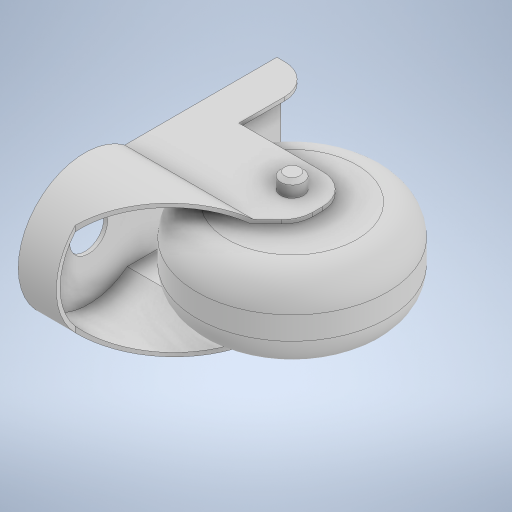
# Autodesk Inventor part: Колесо
Saved by Autodesk Inventor 2023 (Build 270158000, 158)
## iProperties
Created: 2022-04-27
Part Number: Колесо
Material: Типовые
Document SubType Name: Modeling
Designer: User
Density: 1 g/cm^3
Appearance: По умолчанию
Author: User
Autodesk Inventor part; units mm, degrees
ref_plane "YZ Plane" through (0, 0, 0) normal (1, 0, 0) x (0, 1, 0)
sketch "Эскиз1" plane through (0, 0, 0) normal (0, 1, 0) x (-1, 0, 0)
  point P0 (0, 0)
sketch "Эскиз2" plane through (0, 0, 0) normal (0, 1, 0) x (-1, 0, 0)
  line L0 (0, 0) -> (0, -68)
  line L1 (0, -68) -> (-10, -68)
  line L2 (-10, -68) -> (-10, -48)
  line L3 (-10, -48) -> (-40, -48)
  line L4 (0, 0) -> (-10, 0)
  line L5 (-10, 0) -> (-10, -5)
  line L6 (-40, -48) -> (-40, -34)
  line L7 (-40, -34) -> (-10, -5)
  dimension "d0" = 68
  dimension "d1" = 10
  dimension "d2" = 20
  dimension "d3" = 30
  dimension "d4" = 5
  dimension "d5" = 14
  constraints: 16 end point, 3 perpendicular, 2 parallel, 2 point on line, 1 vertical
  measures "d0" distance of L0.start L0.end
  measures "d1" distance of L0.end L1.end
  measures "d2" distance of L1.end L2.end
  measures "d3" distance of L2.end L3.end
  measures "d4" distance of L4.end L5.end
  measures "d5" distance of L3.end L6.end
extrude "Выдавливание1" add sketch "Эскиз2" along normal blind 28
sketch "Эскиз3" plane through (0, 0, -68) normal (-1, 0, 0) x (0, 0, 1)
  line L0 (68, 0) -> (68, 28) projected
  line L1 (68, 14) -> (33, 14)
  arc A0 (40, 0) -> (40, 28) centre (50.5, 14) ccw
  line L2 (0, 0) -> (68, 0) projected
  line L3 (40, 0) -> (0, 0)
  line L4 (20, 28) -> (0, 28) projected
  line L5 (0, 0) -> (0, 28)
  line L6 (0, 28) -> (40, 28)
  line L7 (0, 28) -> (68, 28) projected
  dimension "d8" = 35
  constraints: 8 end point, 3 point on circle, 2 midpoint, 2 point on line, 1 centre point, 1 collinear, 1 horizontal, 1 perpendicular
  measures "d8" distance of L1.start L1.end
extrude "Выдавливание2" add sketch "Эскиз3" against normal blind 40 contours A0 L2 L5 L4 L6 L7 | A0 L2 | L7 A0
ref_plane "РабПлоскость1" through (0, -23.25, 0) normal (0, -1, 0) x (1, 0, 0)
sketch "Эскиз4" plane through (0, -23.25, 0) normal (0, -1, 0) x (1, 0, 0)
  line L0 (0, -68) -> (40, -68) projected
  line L1 (0, -68) -> (10, -68)
  line L2 (10, -68) -> (10, -48)
  line L3 (10, -48) -> (40, -48)
  line L4 (40, -48) -> (40, -34)
  line L5 (10, 0) -> (10, -5) projected
  line L6 (40, -34) -> (10, -5)
  line L7 (0, 0) -> (10, 0) projected
  line L8 (10, -5) -> (10, 0)
  line L9 (10, 0) -> (0, 0)
  line L10 (0, 0) -> (0, -68)
  dimension "d12" = 10
  dimension "d13" = 20
  dimension "d14" = 30
  dimension "d15" = 14
  constraints: 16 end point, 6 perpendicular, 1 point on line
  measures "d12" distance of L0.start L1.end
  measures "d13" distance of L1.end L2.end
  measures "d14" distance of L2.end L3.end
  measures "d15" distance of L3.end L4.end
extrude "Выдавливание3" cut sketch "Эскиз4" against normal blind 139 keep common part
sketch "Эскиз5" plane through (0, 0, 0) normal (-1, 0, 0) x (0, 0, 1)
  arc A0 (-28, 0) -> (-7, 0) centre (-17.5, 14) ccw projected
  circle A1 centre (-17.5, 14) radius 17.5
  line L0 (-68, 0) -> (-68, 28) projected
  line L1 (-28, 0) -> (-68, 0)
  line L2 (-68, 0) -> (-68, 28)
  arc A2 (-7, 28) -> (-28, 28) centre (-17.5, 14) ccw projected
  line L3 (-68, 28) -> (-28, 28)
  point P0 (0, 0)
  constraints: 6 end point, 3 perpendicular, 1 centre point, 1 coincident, 1 point on circle
extrude "Выдавливание4" cut sketch "Эскиз5" against normal blind 43.75 keep common part
sketch "Эскиз6" plane through (40, 0, -34) normal (1, 0, 0) x (0, 0, -1)
  arc A0 (-29, 1.7526) -> (-6, 0) centre (-16.5, 14) ccw projected
  circle A1 centre (-16.5, 14) radius 16.5
  line L0 (0, 0) -> (0, 28) projected
  line L1 (0, 14) -> (34.1975, 14)
  line L2 (34, 28) -> (-6, 28) projected
  line L3 (34, 0) -> (-6, 0) projected
  line L4 (34, 28) -> (34, 0)
  line L5 (34, 0) -> (34, 28) projected
  line L6 (34, 28) -> (34, 27)
  line L7 (34, 27) -> (-6.3388, 27)
  line L8 (34, 0) -> (34, 1)
  line L9 (34, 1) -> (-6.3388, 1)
  line L10 (34, 27) -> (-6.3388, 27)
  line L11 (34, 27) -> (34, 1)
  point P0 (-34, 0)
  point P1 (0, 27)
  dimension "d20" = 33
  dimension "d21" = 1
  dimension "d22" = 1
  constraints: 16 end point, 3 perpendicular, 2 horizontal, 2 point on circle, 2 point on line, 1 centre point, 1 coincident, 1 midpoint
  measures "d20" diameter of A1
  measures "d21" distance of L2.start L6.end
  measures "d22" distance of L3.start L8.end
extrude "Выдавливание5" cut sketch "Эскиз6" against normal blind 39 contours A1 | L0 L9 A1 | L1 L4 L9 L0 | A1 L7 L0 | L0 L7 L4 L1
fillet "Сопряжение1" radius 8 2 edges at (40, 0.5, -48) (40, 27.5, -48)
fillet "Сопряжение2" radius 8 2 edges at (40, 0.5, -34) (40, 27.5, -34)
fillet "Сопряжение3" radius 8 2 edges at (10, 0.5, -68) (10, 27.5, -68)
sketch "Эскиз7" plane through (0, 28, 0) normal (0, 1, 0) x (1, 0, 0)
  arc A0 (40, 40) -> (32, 48) centre (32, 40) ccw projected
  circle A1 centre (32, 40) radius 3
  point P0 (0, 0)
  dimension "d28" = 6
  constraints: 1 centre point, 1 coincident
  measures "d28" diameter of A1
extrude "Выдавливание6" add sketch "Эскиз7" along normal blind 4 and the other way blind 32
sketch "Эскиз8" plane through (1, 0, -34) normal (1, 0, 0) x (0, 0, -1)
  arc A0 (-6.3388, 27) -> (-29, 24.7703) centre (-16.5, 14) ccw projected
  circle A1 centre (-16.5, 14) radius 5
  point P0 (-34, 0)
  dimension "d31" = 10
  constraints: 1 centre point, 1 coincident
  measures "d31" diameter of A1
extrude "Выдавливание7" cut sketch "Эскиз8" against normal blind 31
ref_plane "РабПлоскость2" through (1, 3, -27.6612) normal (0, 1, 0) x (1, 0, 0)
sketch "Эскиз9" plane through (1, 3, -27.6612) normal (0, 1, 0) x (1, 0, 0)
  circle A0 centre (31, 12.3388) radius 3 projected
  circle A1 centre (31, 12.3388) radius 25
  point P0 (-1, -27.6612)
  dimension "d35" = 50
  constraints: 1 centre point, 1 coincident
  measures "d35" diameter of A1
extrude "Выдавливание8" add sketch "Эскиз9" along normal blind 22
fillet "Сопряжение4" radius 8 2 edges at (7, 3, -40) (7, 25, -40)
chamfer "Фаска1" distance 1 angle 45 2 edges at (29, -4, -40) (29, 32, -40)
